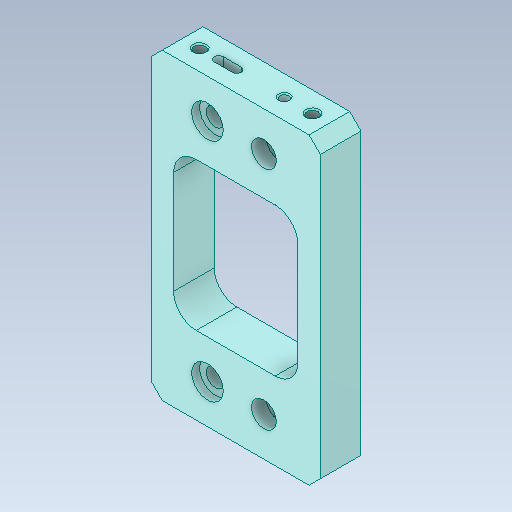
# Autodesk Inventor part: FAB-P0003
Saved by Autodesk Inventor 2020 (Build 240168000, 168)
## iProperties
Created: 2012-05-14
Part Number: FAB-P0003
Material: SolidWorks Materials|6061-T6 (SS)
Description: Support bracket
Document SubType Name: Modeling
Designer: map
Density: 2.7 g/cm^3
Appearance: 192,255,255
Mass: 297.777 g
Surface Area: 280.089 cm^2
Volume: 110.288 cm^3
Company: RESOLUTION DEVELOPMENT SERVICES
Sending System: SolidWorks 2015
Last Author: yl862
Last Saved: 2016-08-08
Author: map
Revision Number: 03
Autodesk Inventor part; units mm, degrees
ref_plane "YZ Plane" through (0, 0, 0) normal (1, 0, 0) x (0, 1, 0)
ref_plane "XZ Plane" through (0, 0, 0) normal (0, 1, 0) x (-1, 0, 0)
ref_plane "XY Plane" through (0, 0, 0) normal (0, 0, 1) x (1, 0, 0)
sketch "3H7Slot" plane through (0, 0, 0) normal (0, 0, 1) x (1, 0, 0)
  line L0 (32.4992, 25.6932) -> (32.4992, 24.1932) construction
  line L1 (30.9992, 25.6932) -> (30.9992, 24.1932)
  line L2 (33.9992, 24.1932) -> (33.9992, 25.6932)
  arc A0 (33.9992, 25.6932) -> (30.9992, 25.6932) centre (32.4992, 25.6932) ccw
  arc A1 (30.9992, 24.1932) -> (33.9992, 24.1932) centre (32.4992, 24.1932) ccw
  point P0 (32.4992, 24.6932)
  dimension "d61" = 3
  dimension "d71" = 1.5
  measures "d61" diameter of A1
  measures "d71" distance of L0.end L0.start
sketch "Sketch1" plane through (32.5, -67.2, -9) normal (0, 0, -1) x (-1, 0, 0)
  point P0 (32.5, 67.2)
sketch "Sketch2" plane through (-32.5, -67.2, 9) normal (0, 0, 1) x (1, 0, 0)
  line L0 (-5, 129.4) -> (-5, 5) projected
  line L1 (-5, 5) -> (0, 0) projected
  line L2 (0, 0) -> (65, 0) projected
  line L3 (65, 0) -> (70, 5) projected
  line L4 (70, 129.4) -> (70, 5) projected
  line L5 (70, 129.4) -> (65, 134.4) projected
  line L6 (0, 134.4) -> (65, 134.4) projected
  line L7 (0, 134.4) -> (-5, 129.4) projected
  line L8 (15, 34.4) -> (50, 34.4) projected
  arc A0 (5, 44.4) -> (15, 34.4) centre (15, 44.4) ccw projected
  line L9 (5, 90) -> (5, 44.4) projected
  arc A1 (15, 100) -> (5, 90) centre (15, 90) ccw projected
  line L10 (50, 100) -> (15, 100) projected
  arc A2 (60, 90) -> (50, 100) centre (50, 90) ccw projected
  line L11 (60, 44.4) -> (60, 90) projected
  arc A3 (50, 34.4) -> (60, 44.4) centre (50, 44.4) ccw projected
  circle A4 centre (20, 17.2) radius 5.5 projected
  circle A5 centre (45, 17.2) radius 5.5 projected
  circle A6 centre (45, 117.2) radius 5.5 projected
  circle A7 centre (20, 117.2) radius 5.5 projected
  circle A8 centre (32.497, 129.748) radius 2 projected
  arc A9 (34.497, 121.251) -> (30.497, 121.251) centre (32.497, 121.251) ccw projected
  line L12 (30.497, 113.251) -> (30.497, 121.251) projected
  arc A10 (30.497, 113.251) -> (34.497, 113.251) centre (32.497, 113.251) ccw projected
  line L13 (34.497, 121.251) -> (34.497, 113.251) projected
  point P0 (32.5, 67.2)
sketch "Sketch3" plane through (-32.5, 67.2, -9) normal (0, 1, 0) x (1, 0, 0)
  line L0 (65, 0) -> (0, 0) projected
  line L1 (0, 0) -> (0, -18) projected
  line L2 (0, -18) -> (65, -18) projected
  line L3 (65, -18) -> (65, 0) projected
  circle A0 centre (7.5, -9) radius 3.5 projected
  circle A1 centre (57.5, -9) radius 3.5 projected
  arc A2 (24, -11) -> (24, -7) centre (24, -9) ccw projected
  line L4 (16, -11) -> (24, -11) projected
  arc A3 (16, -7) -> (16, -11) centre (16, -9) ccw projected
  line L5 (24, -7) -> (16, -7) projected
  circle A4 centre (45, -9) radius 2 projected
  point P0 (32.5, -9)
sketch "Sketch4" plane through (-32.5, -67.2, 9) normal (0, -1, 0) x (1, 0, 0)
  line L0 (0, 0) -> (65, 0) projected
  line L1 (0, 0) -> (0, -18) projected
  line L2 (65, -18) -> (0, -18) projected
  line L3 (65, -18) -> (65, 0) projected
  circle A0 centre (45, -9) radius 2 projected
  line L4 (16, -11) -> (24, -11) projected
  arc A1 (16, -7) -> (16, -11) centre (16, -9) ccw projected
  line L5 (24, -7) -> (16, -7) projected
  arc A2 (24, -11) -> (24, -7) centre (24, -9) ccw projected
  circle A3 centre (57.5, -9) radius 3.5 projected
  circle A4 centre (7.5, -9) radius 3.5 projected
  point P0 (32.5, -9)
extrude "Extrusion1" add sketch "Sketch2" against normal up to surface (18 mm away) from surface at 0 contours L7 L6 L5 L4 L3 L2 L1 L0 | A4 | A5 | A6 | A7 | A8 | L13 A10 L12 A9
hole "M6Clearance" at (12.5, -50, 9) at (12.5, 50, 9) direction (0, 0, -1) diameter 6.6 end through all counterbore diameter 11 counterbore depth 6.5 clearance for "Socket Head Cap Screw ISO 4762" size "M6" standard "ISO"
hole "M6TapsTop" at (25, 67.2, 0) at (-25, 67.2, 0) direction (0, -1, 0) diameter 4.917 depth 17.1 tip angle 118 countersink diameter 6 countersink angle 90 thread size "M6x1" class "6H" standard "ISO Metric profile"
hole "M6TapsBottom" at (25, -67.2, 0) at (-25, -67.2, 0) direction (0, 1, 0) diameter 4.917 depth 17.1 tip angle 118 countersink diameter 6 countersink angle 90 thread size "M6x1" class "6H" standard "ISO Metric profile"
extrude "4H7AlignmentSlot1" cut sketch "Sketch3" against normal blind 8 contours L4 A3 L5 A2
extrude "4H7AlignmentSlot2" cut sketch "Sketch4" against normal blind 8 contours A1 L5 A2 L4
hole "4H7AlignmentHole1" at (12.5, -67.2, 0) direction (0, 1, 0) diameter 4 depth 8 tip angle 118 countersink diameter 5 countersink angle 90
hole "4H7AlignmentHole2" at (12.5, 67.2, 0) direction (0, -1, 0) diameter 4 depth 8 tip angle 118 countersink diameter 5 countersink angle 90
hole "ShoulderScrewHoles" at (-12.5, 50, 9) at (-12.5, -50, 9) direction (0, 0, -1) diameter 8 end through all counterbore diameter 14 counterbore depth 3.5
body "Solid1"
